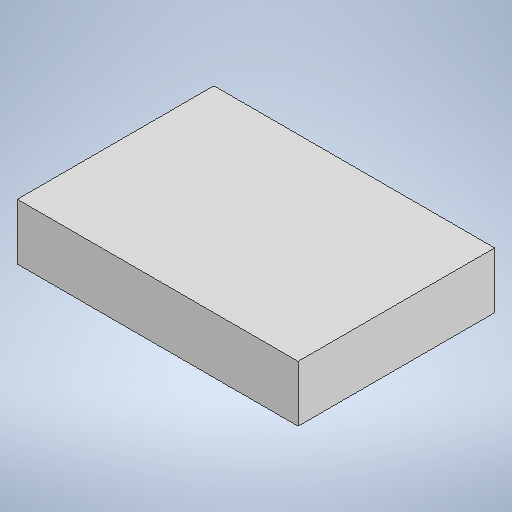
# Autodesk Inventor part: Small_Sensor
Saved by Autodesk Inventor 2027 (Build 310192000, 192)
## iProperties
Created: 2026-09-10
Part Number: Small_Sensor
Material: Generic
Document SubType Name: Modeling
Designer: IG2
Density: 1 g/cm^3
Appearance: Default
Author: IG2
Autodesk Inventor part; units mm, degrees
ref_plane "YZ Plane" through (0, 0, 0) normal (1, 0, 0) x (0, 1, 0)
ref_plane "XZ Plane" through (0, 0, 0) normal (0, 1, 0) x (-1, 0, 0)
ref_plane "XY Plane" through (0, 0, 0) normal (0, 0, 1) x (1, 0, 0)
sketch "Sketch1" plane through (0, 0, 0) normal (0, 0, 1) x (1, 0, 0)
  line L0 (-50, -13.142) -> (50, -13.142)
  line L1 (50, -13.142) -> (50, 6.858)
  line L2 (50, 6.858) -> (-50, 6.858)
  line L3 (-50, 6.858) -> (-50, -13.142)
  line L4 (0, 6.858) -> (0, 0)
  dimension "d0" = 50
  dimension "d1" = 20
  constraints: 10 end point, 2 parallel, 1 horizontal, 1 midpoint, 1 perpendicular, 1 vertical
  measures "d0" distance between parallel lines of L1 L4
  measures "d1" distance between parallel lines of L0 L2
extrude "Extrusion1" add sketch "Sketch1" along normal mid plane 70
body "Solid1"
